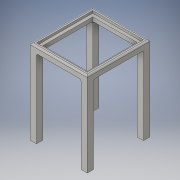
# Autodesk Inventor part: Hood_base
Saved by Autodesk Inventor 2016 (Build 200138000, 138)
## iProperties
Created: 2018-09-18
Part Number: Hood_base
Material: Generic
Document SubType Name: Modeling
Designer: Kyle
Density: 1 g/cm^3
Appearance: Default
Author: Kyle
Autodesk Inventor part; units mm, degrees
ref_plane "YZ Plane" through (0, 0, 0) normal (1, 0, 0) x (0, 1, 0)
ref_plane "XZ Plane" through (0, 0, 0) normal (0, 1, 0) x (-1, 0, 0)
ref_plane "XY Plane" through (0, 0, 0) normal (0, 0, 1) x (1, 0, 0)
sketch "Sketch1" plane through (0, 0, 0) normal (0, 1, 0) x (-1, 0, 0)
  line L0 (-36.5, -40) -> (-36.5, 40)
  line L1 (36.5, 40) -> (36.5, -40)
  line L2 (-36.5, 40) -> (36.5, -40) construction
  line L3 (36.5, 40) -> (-36.5, -40) construction
  line L4 (36.5, 40) -> (36.5, 13)
  line L5 (-36.5, 40) -> (36.5, 40)
  line L6 (-36.5, -40) -> (-9.5, -40)
  line L7 (-36.5, -40) -> (18.5, -40)
  line L8 (36.5, -40) -> (-36.5, -40)
  line L9 (36.5, -40) -> (28.5, -40)
  line L10 (28.5, -40) -> (28.5, -32)
  line L11 (28.5, -32) -> (36.5, -32)
  line L12 (36.5, -32) -> (36.5, -40)
  line L13 (36.5, 40) -> (28.5, 40)
  line L14 (28.5, 40) -> (28.5, 32)
  line L15 (28.5, 32) -> (36.5, 32)
  line L16 (36.5, 32) -> (36.5, 40)
  line L17 (-36.5, 40) -> (-28.5, 40)
  line L18 (-28.5, 40) -> (-28.5, 32)
  line L19 (-28.5, 32) -> (-36.5, 32)
  line L20 (-36.5, 32) -> (-36.5, 40)
  line L21 (-36.5, -40) -> (-28.5, -40)
  line L22 (-28.5, -40) -> (-28.5, -32)
  line L23 (-28.5, -32) -> (-36.5, -32)
  line L24 (-36.5, -32) -> (-36.5, -40)
  dimension "d0" = 73
  dimension "d1" = 80
  dimension "d10" = 8
  dimension "d11" = 8
  dimension "d12" = 8
  dimension "d13" = 8
  dimension "d14" = 8
  dimension "d15" = 8
  dimension "d16" = 8
  dimension "d17" = 8
  constraints: 50 end point, 10 parallel, 6 horizontal, 5 perpendicular, 3 point on line, 1 vertical
  measures "d0" distance of L8.start L8.end
  measures "d1" distance of L1.start L8.start
  measures "d10" distance of L10.end L11.end
  measures "d11" distance of L9.end L10.end
  measures "d12" distance of L15.end L14.end
  measures "d13" distance of L14.end L13.end
  measures "d14" distance of L18.end L19.end
  measures "d15" distance of L17.end L18.end
  measures "d16" distance of L23.end L22.end
  measures "d17" distance of L22.end L21.end
extrude "Extrusion1" add sketch "Sketch1" along normal blind 100 contours L0 L23 L22 L6 | L0 L5 L18 L19 | L10 L11 L1 L8 | L5 L1 L15 L14
sketch "Sketch2" plane through (0, 100, 0) normal (0, 1, 0) x (1, 0, 0)
  line L0 (-36.5, -40) -> (-28.5, -40) projected
  line L1 (-28.5, 32) -> (-28.5, 40) projected
  line L2 (-36.5, -40) -> (-28.5, -40)
  line L3 (-28.5, -40) -> (-28.5, 40)
  line L4 (-28.5, 40) -> (-36.5, 40)
  line L5 (-36.5, 40) -> (-36.5, -40)
  line L6 (-36.5, -32) -> (-36.5, -40) projected
  line L7 (36.5, -40) -> (36.5, -32) projected
  line L8 (-36.5, -40) -> (36.5, -40)
  line L9 (36.5, -40) -> (36.5, -32)
  line L10 (36.5, -32) -> (-36.5, -32)
  line L11 (-36.5, -32) -> (-36.5, -40)
  line L12 (28.5, -32) -> (28.5, -40) projected
  line L13 (36.5, 40) -> (28.5, 40) projected
  line L14 (28.5, -32) -> (36.5, -32)
  line L15 (36.5, -32) -> (36.5, 40)
  line L16 (36.5, 40) -> (28.5, 40)
  line L17 (28.5, 40) -> (28.5, -32)
  line L18 (-28.5, 32) -> (-28.5, 40) projected
  line L19 (28.5, 40) -> (28.5, 32) projected
  line L20 (-28.5, 40) -> (28.5, 40)
  line L21 (28.5, 40) -> (28.5, 32)
  line L22 (28.5, 32) -> (-28.5, 32)
  line L23 (-28.5, 32) -> (-28.5, 40)
  point P0 (0, 0)
  constraints: 32 end point, 8 parallel, 4 horizontal, 4 perpendicular
extrude "Extrusion2" add sketch "Sketch2" along normal blind 8 contours L5 L10 L3 L0 | L3 L10 L12 L8 | L5 L4 L1 L3 L10 | L12 L10 L7 L8 | L1 L20 L17 L22 | L17 L13 L15 L10
sketch "Sketch3" plane through (0, 108, 0) normal (0, 1, 0) x (1, 0, 0)
  line L0 (28.5, -32) -> (-28.5, -32) projected
  line L1 (28.5, 32) -> (36.5, 32) projected
  line L2 (-28.5, -32) -> (28.5, -32)
  line L3 (28.5, -32) -> (28.5, 32)
  line L4 (28.5, 32) -> (-28.5, 32)
  line L5 (-28.5, 32) -> (-28.5, -32)
  line L6 (32.5, 36) -> (32.5, -36)
  line L7 (32.5, -36) -> (-32.5, -36)
  line L8 (-32.5, -36) -> (-32.5, 36)
  line L9 (-32.5, 36) -> (32.5, 36)
  point P0 (0, 0)
  dimension "d22" = 4
  constraints: 16 end point, 4 parallel, 2 perpendicular, 1 horizontal, 3 other
  measures "d22" distance between parallel lines of L3 L6
extrude "Extrusion3" cut sketch "Sketch3" against normal blind 3
fillet "Fillet1" radius 2 8 edges at (32.5, 100, 32) (-28.5, 100, -36) (-28.5, 100, 36) (28.5, 100, -36) (-32.5, 100, 32) (-32.5, 100, -32) (28.5, 100, 36) (32.5, 100, -32)
fillet "Fillet2" radius 2 4 edges at (-36.5, 108, 0) (0, 108, 40) (36.5, 108, 0) (0, 108, -40)
body "Solid1"
